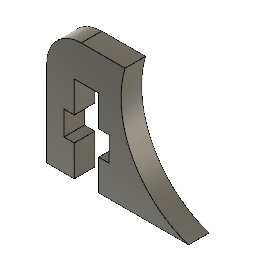
stator_mount v4 (Autodesk Fusion 360 design; units mm, degrees)
Autodesk Fusion 360 part; units mm, degrees
sketch "Sketch1" plane through (0, 0, 0) normal (0, 1, 0) x (1, 0, 0)
  circle A0 centre (0, 0) radius 28.5
  line L0 (-9, 27.0416) -> (9, 27.0416)
  line L1 (-27.3663, -7.9584) -> (-40, -7.9584)
  line L2 (-50, 2.0416) -> (-50, 27.0416)
  line L3 (-50, 27.0416) -> (-9, 27.0416)
  line L4 (-42, 27.0416) -> (-35, 27.0416)
  line L5 (-35, 27.0416) -> (-35, 2.0416)
  line L6 (-35, 2.0416) -> (-42, 2.0416)
  line L7 (-42, 2.0416) -> (-42, 27.0416)
  line L8 (-42, 2.0416) -> (-50, 2.0416)
  line L9 (-50, 2.0416) -> (-35, 2.0416)
  line L10 (-28.4268, 2.0416) -> (-35, 2.0416)
  line L11 (-45, 11.0416) -> (-32, 11.0416)
  line L12 (-32, 11.0416) -> (-32, 18.0416)
  line L13 (-32, 18.0416) -> (-45, 18.0416)
  line L14 (-45, 18.0416) -> (-45, 11.0416)
  line L15 (-38.5, 18.0416) -> (-38.5, 27.0416)
  line L16 (-45, 14.5416) -> (-42, 14.5416)
  line L17 (-45, 11.0416) -> (-50, 11.0416)
  line L18 (-32, 11.0416) -> (-26.2742, 11.0416)
  arc A1 (-50, 2.0416) -> (-40, -7.9584) centre (-40, 2.0416) ccw
  line L19 (0, 27.0416) -> (0, 0)
  line L20 (27.3663, -7.9584) -> (40, -7.9584)
  arc A2 (40, -7.9584) -> (50, 2.0416) centre (40, 2.0416) ccw
  line L21 (50, 2.0416) -> (50, 27.0416)
  line L22 (50, 27.0416) -> (9, 27.0416)
  line L23 (32, 18.0416) -> (45, 18.0416)
  line L24 (32, 11.0416) -> (32, 18.0416)
  line L25 (45, 11.0416) -> (32, 11.0416)
  line L26 (45, 18.0416) -> (45, 11.0416)
  line L27 (42, 2.0416) -> (42, 27.0416)
  line L28 (35, 27.0416) -> (35, 2.0416)
  line L29 (35, 2.0416) -> (42, 2.0416)
  line L30 (-50, 11.0416) -> (-26.2742, 11.0416)
  dimension "d1" = 57
  dimension "d2" = 18
  dimension "d3" = 25
  dimension "d4" = 90
  dimension "d5" = 10
  dimension "d8" = 7
  dimension "d9" = 7
  dimension "d10" = 13
  dimension "d11" = 90
  dimension "d12" = 90
  dimension "d15" = 10
  dimension "d22" = 100
  dimension "d23" = 5
  constraint coincident A0.centre L19.end
  constraint coincident A0 L0.start
  constraint coincident A0 L0.end
  constraint horizontal L0
  constraint coincident A0 L1.start
  constraint perpendicular L0 L2
  constraint perpendicular L2 L3
  constraint horizontal L4
  constraint vertical L5
  constraint horizontal L6
  constraint vertical L7
  constraint coincident L3 L4.start
  constraint coincident L2 L8.end
  constraint perpendicular L2 L8
  constraint perpendicular L5 L9
  constraint coincident A0 L10.start
  constraint perpendicular L5 L10
  constraint horizontal L11
  constraint vertical L12
  constraint horizontal L13
  constraint vertical L14
  constraint midpoint L13 L15.start
  constraint midpoint L4 L15.end
  constraint midpoint L14 L16.start
  constraint midpoint L7 L16.end
  constraint perpendicular L2 L17
  constraint coincident A0 L18.end
  constraint perpendicular L12 L18
  constraint coincident L2 L17.end
  constraint tangent L1 A1
  constraint tangent L2 A1
  constraint midpoint L0 L19.start
  constraint symmetric L0.start L19 L0.end
  constraint symmetric L1.start L19 L20.start
  constraint symmetric L2.end L19 L21.end
  constraint symmetric L4.start L19 L27.end
  constraint symmetric L4.end L19 L28.start
  constraint symmetric L5.end L19 L28.end
  constraint symmetric L6.end L19 L27.start
  constraint symmetric L11.start L19 L25.start
  constraint symmetric L11.end L19 L24.start
  constraint symmetric L12.end L19 L23.start
  constraint symmetric L13.end L19 L23.end
  constraint symmetric L1.end L19 L20.end
  constraint symmetric L2.start L19 A2.end
  constraint symmetric A1 L19 A2
  measures "d1" diameter of A0
  measures "d2" distance of L0.start L0.end
  measures "d3" distance of L4.end L5.end
  measures "d4" angle of L1 L2
  measures "d5" distance of L1 L6
  measures "d8" distance of L5 L7
  measures "d9" distance of L11.start L13.end
  measures "d10" distance of L12 L14
  measures "d11" angle of L7 L16
  measures "d12" angle of L4 L15
  measures "d15" radius of A1
  measures "d22" distance of L2 L21
  measures "d23" distance of L11.start L17.end
extrude "Extrude1" add sketch "Sketch1" along normal blind 5 contours A0 L20 A2 L21 L22 L23 L24 L25 L26 L27 L28 L29 | A0 L3 L5 L12 L13 L18 L30 | A0 L1 L6 L8 L9 L10 A1 | A0 L5 L10 L11 L18 L30 | L2 L7 L8 L9 L11 L17 L30 | L2 L3 L7 L13 L14 L17 L30 makes body 1 at (-34.4021, 5, 3.3326) makes body 2 at (34.4021, 5, 3.3326)
extrude "Extrude2" cut 1 faces at (34.4021, 0, 3.3326) along direction (0, 1, 0) blind 10 on bodies 2 bodies 2
extrude "Extrude3" add 1 faces at (-34.4021, 0, 3.3326) along direction (0, -1, 0) blind 1 on bodies 1 bodies 1 2
